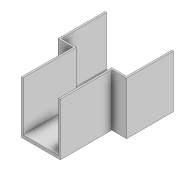
# Autodesk Inventor part: large_room1
Saved by Autodesk Inventor 2021 (Build 250183000, 183)
## iProperties
Created: 2022-05-19
Part Number: large_room1
Material: Generic
Document SubType Name: Modeling
Designer: Derm
Density: 1 g/cm^3
Appearance: Default
Author: Derm
Autodesk Inventor part; units mm, degrees
ref_plane "YZ Plane" through (0, 0, 0) normal (1, 0, 0) x (0, 1, 0)
ref_plane "XZ Plane" through (0, 0, 0) normal (0, 1, 0) x (-1, 0, 0)
ref_plane "XY Plane" through (0, 0, 0) normal (0, 0, 1) x (1, 0, 0)
sketch "Sketch1" plane through (0, 0, 0) normal (0, 1, 0) x (-1, 0, 0)
  line L0 (0, 0) -> (0, -12.8272) construction
  line L1 (9.1218, 27.3958) -> (9.1218, 0)
  line L2 (9.1218, 0) -> (16.7753, 0)
  line L3 (16.7753, 0) -> (16.7753, -23.2516)
  line L4 (10.0041, 27.3958) -> (10.0041, 0.8823)
  line L5 (10.0041, 0.8823) -> (17.6575, 0.8823)
  line L6 (17.6575, 0.8823) -> (17.6575, -23.2516)
  line L7 (10.0041, 27.3958) -> (9.1218, 27.3958)
  line L8 (16.7753, -23.2516) -> (17.6575, -23.2516)
  line L9 (-9.1218, 27.3958) -> (-9.1218, 0)
  line L10 (-9.1218, 0) -> (-16.7753, 0)
  line L11 (-16.7753, 0) -> (-16.7753, -23.2516)
  line L12 (-10.0041, 27.3958) -> (-10.0041, 0.8823)
  line L13 (-10.0041, 0.8823) -> (-17.6575, 0.8823)
  line L14 (-17.6575, 0.8823) -> (-17.6575, -23.2516)
  line L15 (-10.0041, 27.3958) -> (-9.1218, 27.3958)
  line L16 (-16.7753, -23.2516) -> (-17.6575, -23.2516)
  constraints: 34 end point, 8 symmetric about line, 4 perpendicular, 2 horizontal, 2 vertical, 2 other
extrude "Extrusion1" add sketch "Sketch1" against normal mid plane 25.4
sketch "Sketch2" plane through (0, -12.7, 0) normal (0, -1, 0) x (1, 0, 0)
  line L0 (-9.1218, 0) -> (-9.1218, 27.3958) projected
  line L1 (-9.1218, 27.3958) -> (-10.0041, 27.3958) projected
  line L2 (-10.0041, 27.3958) -> (-10.0041, 0.8823) projected
  line L3 (-10.0041, 0.8823) -> (-17.6575, 0.8823) projected
  line L4 (-17.6575, 0.8823) -> (-17.6575, -23.2516) projected
  line L5 (-17.6575, -23.2516) -> (-16.7753, -23.2516) projected
  line L6 (-16.7753, -23.2516) -> (-16.7753, 0) projected
  line L7 (-16.7753, 0) -> (-9.1218, 0) projected
  line L8 (17.6575, 0.8823) -> (10.0041, 0.8823) projected
  line L9 (10.0041, 0.8823) -> (10.0041, 27.3958) projected
  line L10 (10.0041, 27.3958) -> (9.1218, 27.3958) projected
  line L11 (9.1218, 27.3958) -> (9.1218, 0) projected
  line L12 (9.1218, 0) -> (16.7753, 0) projected
  line L13 (16.7753, 0) -> (16.7753, -23.2516) projected
  line L14 (16.7753, -23.2516) -> (17.6575, -23.2516) projected
  line L15 (17.6575, -23.2516) -> (17.6575, 0.8823) projected
  line L16 (10.0041, 27.3958) -> (9.1218, 27.3958) projected
  line L17 (-9.1218, 27.3958) -> (-10.0041, 27.3958) projected
  line L18 (10.0041, 27.3958) -> (-10.0041, 27.3958)
  line L19 (17.6575, 0.8823) -> (17.6575, -23.2516) projected
  line L20 (17.6575, -23.2516) -> (-17.6575, -23.2516)
  point P0 (0, 0)
  constraints: 4 end point, 1 horizontal, 1 perpendicular
extrude "Extrusion2" add sketch "Sketch2" along normal blind 1.5875
body "Solid1"
